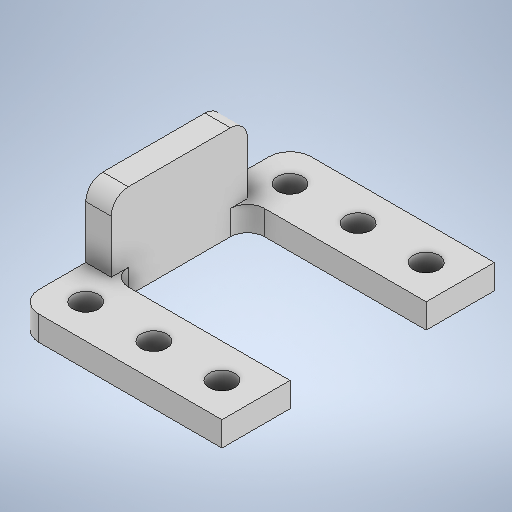
# Autodesk Inventor part: CH-1-03-RearGearboxSpacer_01
Saved by Autodesk Inventor 2025.1 (Build 291241020, 241B)
## iProperties
Created: 2024-10-23
Part Number: CH-1-03-RearGearboxSpacer_01
Material: Generic
Document SubType Name: Modeling
Designer: aidan
Density: 1 g/cm^3
Appearance: Default
Author: aidan
Autodesk Inventor part; units mm, degrees
note: some values were not read from the file. Chosen so that the rebuilt part matches the saved one: edges of "Fillet8".
ref_plane "YZ Plane" through (0, 0, 0) normal (1, 0, 0) x (0, 1, 0)
ref_plane "XZ Plane" through (0, 0, 0) normal (0, 1, 0) x (-1, 0, 0)
ref_plane "XY Plane" through (0, 0, 0) normal (0, 0, 1) x (1, 0, 0)
sketch "Sketch1" plane through (0, 0, 0) normal (1, 0, 0) x (0, 1, 0)
  line L0 (0, 0) -> (9.144, 0)
  line L1 (9.144, 0) -> (9.144, -25.4)
  line L2 (9.144, -25.4) -> (0, -25.4)
  line L3 (0, -25.4) -> (0, 0)
  dimension "d0" = 25.4
  dimension "d1" = 9.144
  constraints: 8 end point, 2 parallel, 1 horizontal, 1 perpendicular
  measures "d0" distance of L2.end L0.start
  measures "d1" distance of L1.end L2.end
extrude "Extrusion1" add sketch "Sketch1" along normal blind 63.5
sketch "Sketch2" plane through (0, 9.144, 0) normal (0, 1, 0) x (1, 0, 0)
  line L0 (0, 25.4) -> (0, 0) projected
  line L1 (0, 12.7) -> (6.35, 12.7)
  line L2 (6.35, 12.7) -> (31.75, 12.7)
  line L3 (31.75, 12.7) -> (57.15, 12.7)
  circle A0 centre (6.35, 12.7) radius 4.7625
  circle A1 centre (31.75, 12.7) radius 4.7625
  circle A2 centre (57.15, 12.7) radius 4.7625
  dimension "d4" = 6.35
  dimension "d5" = 25.4
  dimension "d6" = 25.4
  dimension "d7" = 9.525
  dimension "d8" = 9.525
  dimension "d9" = 9.525
  constraints: 6 end point, 3 centre point, 3 coincident, 2 point on line, 1 horizontal, 1 midpoint
  measures "d4" distance of L1.start L1.end
  measures "d5" distance of L1.end L2.end
  measures "d6" distance of L2.end L3.end
  measures "d7" diameter of A0
  measures "d8" diameter of A1
  measures "d9" diameter of A2
sketch "Sketch3" plane through (0, 0, 0) normal (-1, 0, 0) x (0, 0, 1)
  line L0 (-25.4, 0) -> (-25.4, 9.144) projected
  line L1 (0, 0) -> (-25.4, 0)
  line L2 (-25.4, 0) -> (-25.4, 9.144)
  line L3 (-25.4, 9.144) -> (0, 9.144)
  line L4 (0, 9.144) -> (0, 0)
  constraints: 8 end point, 2 parallel, 1 horizontal, 1 perpendicular
extrude "Extrusion2" add sketch "Sketch3" along normal blind 3.175
extrude "Extrusion3" cut sketch "Sketch2" against normal blind 25.4
sketch "Sketch4" plane through (63.5, 0, 0) normal (1, 0, 0) x (0, 0, -1)
  line L0 (25.4, 0) -> (25.4, 9.144) projected
  line L1 (25.4, 9.144) -> (0, 9.144) projected
  line L2 (0, 9.144) -> (0, 0) projected
  line L3 (0, 0) -> (25.4, 0) projected
extrude "Extrusion4" add sketch "Sketch4" along normal blind 5.08
sketch "Sketch5" plane through (68.58, 0, 0) normal (1, 0, 0) x (0, 0, -1)
  line L0 (25.4, 9.144) -> (0, 9.144) projected
  line L1 (0, 9.144) -> (0, 0) projected
  line L2 (0, 0) -> (25.4, 0) projected
  line L3 (25.4, 0) -> (25.4, 9.144) projected
extrude "Extrusion5" add sketch "Sketch5" along normal blind 1.27
sketch "Sketch8" plane through (-3.175, 0, -25.4) normal (0, 0, -1) x (-1, 0, 0)
  line L0 (-73.025, 0) -> (0, 0) projected
  line L1 (0, 9.144) -> (-73.025, 9.144) projected
  line L2 (0, 0) -> (-15.875, 0)
  line L3 (-15.875, 0) -> (-15.875, 9.144)
  line L4 (-15.875, 9.144) -> (0, 9.144)
  line L5 (0, 9.144) -> (0, 0)
  line L6 (0, 9.144) -> (0, 0) projected
  point P0 (-3.175, 0)
  point P1 (0, 4.572)
  dimension "d24" = 15.875
  constraints: 8 end point, 2 parallel, 1 horizontal, 1 midpoint, 1 perpendicular, 1 point on line
  measures "d24" distance from line of point (0, 4.572) L3
extrude "Extrusion8" add sketch "Sketch8" along normal blind 50.8
sketch "Sketch9" plane through (-3.175, 0, 0) normal (-1, 0, 0) x (0, 0, 1)
  line L0 (0, 0) -> (0, 9.144) projected
  line L1 (0, 9.144) -> (-76.2, 9.144) projected
  line L2 (-76.2, 0) -> (-76.2, 9.144) projected
  line L3 (0, 0) -> (-76.2, 0) projected
extrude "Extrusion9" add sketch "Sketch9" along normal blind 3.175
sketch "Sketch10" plane through (69.85, 9.144, 0) normal (0, 1, 0) x (1, 0, 0)
  line L0 (-57.15, 25.4) -> (-57.15, 76.2) projected
  line L1 (-57.15, 76.2) -> (-66.675, 76.2)
  line L2 (-57.15, 76.2) -> (-76.2, 76.2) projected
  line L3 (-71.4375, 41.2761) -> (-61.9125, 41.2761)
  line L4 (-71.4375, 60.3261) -> (-61.9125, 60.3261)
  circle A0 centre (-66.675, 41.2761) radius 4.7625
  circle A1 centre (-66.675, 60.3261) radius 4.7625
  line L5 (-71.4375, 41.2761) -> (-71.4375, 60.3261)
  line L6 (-61.9125, 60.3261) -> (-61.9125, 41.2761)
  point P0 (-69.85, 0)
  dimension "d55" = 9.525
  dimension "d29" = 9.525
  dimension "d56" = 9.525
  constraints: 10 end point, 3 midpoint, 2 point on circle, 1 centre point, 1 parallel, 1 vertical, 3 other
  measures "d29" distance of L0.end L1.end
  measures "d56" diameter of A1
extrude "Extrusion10" add sketch "Sketch10" along normal blind 35.179
sketch "Sketch11" plane through (-3.175, 0, -76.2) normal (0, 0, -1) x (-1, 0, 0)
  line L0 (-15.875, 9.144) -> (3.175, 9.144) projected
  line L1 (-15.875, 9.144) -> (-15.875, 0) projected
  line L2 (-15.875, 0) -> (3.175, 0) projected
  line L3 (3.175, 9.144) -> (3.175, 0) projected
  point P0 (-3.175, 0)
extrude "Extrusion11" add sketch "Sketch11" along normal blind 25.4
sketch "Sketch13" plane through (12.7, 0, -25.4) normal (1, 0, 0) x (0, 0, -1)
  line L0 (0, 9.144) -> (76.2, 9.144) projected
  line L1 (-25.4, 0) -> (76.2, 0) projected
  line L2 (76.2, 9.144) -> (50.8, 9.144)
  line L3 (50.8, 9.144) -> (50.8, 0)
  line L4 (50.8, 0) -> (76.2, 0)
  line L5 (76.2, 0) -> (76.2, 9.144)
  dimension "d38" = 25.4
  constraints: 8 end point, 2 parallel, 1 horizontal, 1 perpendicular, 1 point on line
  measures "d38" distance of L4.end L3.end
extrude "Extrusion12" add sketch "Sketch13" along normal blind 57.15
sketch "Sketch14" plane through (69.85, 9.144, 0) normal (0, 1, 0) x (1, 0, 0)
  circle A0 centre (-12.7, 12.7) radius 4.7625 projected
  line L0 (-12.7, 12.7) -> (-12.7, 88.9)
  circle A1 centre (-38.1, 12.7) radius 4.7625 projected
  line L1 (-38.1, 12.7) -> (-38.1, 88.9)
  circle A2 centre (-12.7, 88.9) radius 4.7625
  circle A3 centre (-38.1, 88.9) radius 4.7625
  circle A4 centre (-63.5, 12.7) radius 4.7625 projected
  line L2 (-63.5, 12.7) -> (-63.5, 88.9)
  circle A5 centre (-63.5, 88.9) radius 4.7625
  point P0 (-69.85, 0)
  dimension "d42" = 76.2
  dimension "d43" = 76.2
  dimension "d44" = 9.525
  dimension "d45" = 9.525
  dimension "d46" = 9.525
  constraints: 6 end point, 3 centre point, 3 coincident, 3 vertical
  measures "d42" distance of L0.start L0.end
  measures "d43" distance of L1.start L1.end
  measures "d44" diameter of A2
  measures "d45" diameter of A3
  measures "d46" diameter of A5
extrude "Extrusion13" cut sketch "Sketch14" against normal blind 20.6375 contours A2 | A3 | A5
fillet "Fillet2" radius 7.9375 2 edges at (-6.35, 4.572, -101.6) (-6.35, 4.572, 0)
sketch "Sketch15" plane through (69.85, 9.144, 0) normal (0, 1, 0) x (1, 0, 0)
  line L0 (0, 25.4) -> (-57.15, 25.4) projected
  line L1 (-57.15, 25.4) -> (-76.2, 25.4)
  line L2 (-76.2, 7.9375) -> (-76.2, 93.6625) projected
  line L3 (-57.15, 25.4) -> (-57.15, 76.2) projected
  line L4 (-57.15, 76.2) -> (-76.2, 76.2)
  line L5 (-71.4375, 31.7511) -> (-71.4375, 69.8511) projected
  line L6 (-61.9125, 69.8511) -> (-61.9125, 31.7511) projected
  arc A0 (-71.4375, 31.7511) -> (-61.9125, 31.7511) centre (-66.675, 31.7511) ccw projected
  arc A1 (-61.9125, 69.8511) -> (-71.4375, 69.8511) centre (-66.675, 69.8511) ccw projected
  arc A2 (-71.4375, 41.2761) -> (-61.9125, 41.2761) centre (-66.675, 41.2761) ccw projected
  arc A3 (-61.9125, 60.3261) -> (-71.4375, 60.3261) centre (-66.675, 60.3261) ccw projected
  point P0 (-69.85, 0)
  constraints: 4 end point, 2 horizontal, 1 point on line
extrude "Extrusion14" add sketch "Sketch15" along normal blind 26.035 contours L1 L2 L4 L3 | L5 A2 L6 A0 | L5 A1 L6 A3
fillet "Fillet3" radius 6.35 2 edges at (3.175, 35.179, -76.2) (3.175, 35.179, -25.4)
sketch "Sketch16" plane through (-1.5875, 44.323, -60.3261) normal (-1, 0, 0) x (0, 0, 1)
  arc A0 (-9.5239, -9.144) -> (-15.8739, -15.494) centre (-9.5239, -15.494) ccw projected
  line L0 (-9.5239, -9.144) -> (49.3517, -9.144)
  line L1 (49.3517, -9.144) -> (49.3517, 6.1013)
  line L2 (49.3517, 6.1013) -> (-9.5239, 6.1013)
  line L3 (-9.5239, 6.1013) -> (-9.5239, -9.144)
  point P0 (60.3261, -44.323)
  constraints: 8 end point, 2 parallel, 1 horizontal, 1 perpendicular
extrude "Extrusion15" cut sketch "Sketch16" against normal blind 21.971
sketch "Sketch19" plane through (69.85, 35.179, 0) normal (0, 1, 0) x (1, 0, 0)
  line L0 (-57.15, 76.2) -> (-76.2, 76.2) projected
  line L1 (-57.15, 25.4) -> (-76.2, 25.4) projected
  line L2 (-57.15, 76.2) -> (-66.675, 76.2)
  line L3 (-66.675, 76.2) -> (-66.675, 25.4)
  line L4 (-66.675, 25.4) -> (-57.15, 25.4)
  line L5 (-57.15, 25.4) -> (-57.15, 76.2)
  line L6 (-57.15, 76.2) -> (-49.094, 76.2)
  line L7 (-49.094, 76.2) -> (-49.094, 25.4)
  line L8 (-49.094, 25.4) -> (-57.15, 25.4)
  line L9 (-57.15, 25.4) -> (-57.15, 76.2)
  point P0 (-69.85, 0)
  constraints: 16 end point, 4 parallel, 2 horizontal, 2 perpendicular, 1 midpoint, 1 point on line
extrude "Extrusion18" cut sketch "Sketch19" against normal blind 42.8625
fillet "Fillet8" radius 6.35 2 edges at (3.175, 4.572, -76.2) (3.175, 4.572, -25.4)
body "Solid1"
